tripodhook (Autodesk Fusion 360 design; units mm, degrees)
Autodesk Fusion 360 part; units mm, degrees
sketch "Sketch1" plane through (0, 0, 0) normal (0, 0, 1) x (1, 0, 0)
  line L0 (-15, -10) -> (-15, 10)
  line L1 (-15, 10) -> (15, 10)
  line L2 (15, 10) -> (15, -10)
  line L3 (15, -10) -> (-15, 10) construction
  line L4 (-15, -10) -> (15, 10) construction
  line L5 (15, -10) -> (15, -25)
  line L6 (0.0079, -14.5) -> (-15, -14.5)
  line L7 (-15, -10) -> (-15, -14.5)
  arc A0 (-10.5, -25) -> (-0.0079, -14.5) centre (0, -25) ccw
  arc A1 (-15, -25) -> (-10.7121, -14.5) centre (0, -25) ccw
  arc A2 (-10.5, -25) -> (-15, -25) centre (-12.75, -25) ccw
  line L8 (6, 6) -> (-6, 6)
  line L9 (-6, 6) -> (-6, -6)
  line L10 (-6, -6) -> (6, -6)
  line L11 (6, -6) -> (6, 6)
  line L12 (6, 6) -> (-6, -6) construction
  line L13 (-6, 6) -> (6, -6) construction
  circle A3 centre (-11.792, 0) radius 1.75
  circle A4 centre (11.792, 0) radius 1.75
  dimension "d1" = 30
  dimension "d3" = 12
  dimension "d4" = 12
  dimension "d5" = 3.5
  constraint parallel L0 L2
  constraint coincident L3 origin
  constraint coincident L4 origin
  constraint coincident L5.end A1
  constraint tangent L5 A1
  constraint coincident L6.start A0
  constraint horizontal L6
  constraint perpendicular L6 L7
  constraint concentric A0 A1
  constraint coincident L6 A0.end
  constraint coincident L6 A1.end
  constraint tangent A0 A2
  constraint horizontal L8
  constraint perpendicular L8 L9
  constraint parallel L8 L10
  constraint parallel L9 L11
  constraint coincident L12 origin
  constraint coincident L13 origin
  measures "d1" distance of L0.end L1.end
  measures "d3" distance of L9.end L10.end
  measures "d4" distance of L8.end L9.end
  measures "d5" diameter of A3
extrude "Extrude1" add sketch "Sketch1" along normal mid plane 4 contours L0 L1 L2 L5 L6 L7 A1
extrude "Extrude2" add sketch "Sketch1" along normal mid plane 4 contours L6 A0 A1 A2
fillet "Fillet1" radius 4 2 edges at (-15, 10, 0) (15, 10, 0)
fillet "Fillet2" radius 4 1 edges at (-15, -14.5, 0)
fillet "Fillet3" radius 1 20 edges at (13.8284, 8.8284, 2) (0, 10, 2) (-13.8284, 8.8284, 2) (-15, -2.25, 2) (-13.8284, -13.3284, 2) (-5.5039, -14.5, 2) (7.4274, -32.4218, 2) (-12.75, -22.75, 2) (0, -40, 2) (15, -9.5, 2) (7.4274, -32.4218, -2) (-5.5039, -14.5, -2) (-13.8284, -13.3284, -2) (-15, -2.25, -2) (-13.8284, 8.8284, -2) (0, 10, -2) (13.8284, 8.8284, -2) (15, -9.5, -2) (0, -40, -2) (-12.75, -22.75, -2)
